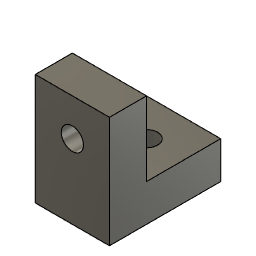
L_1.0 (Autodesk Fusion 360 design; units mm, degrees)
Autodesk Fusion 360 part; units mm, degrees
sketch "Sketch1" plane through (0, 0, 0) normal (0, 1, 0) x (1, 0, 0)
  line L0 (0, 0) -> (10, 0)
  line L1 (5, 0) -> (5, 10)
  line L2 (0, 0) -> (0, 15)
  line L3 (0, 15) -> (10, 15)
  line L4 (10, 15) -> (10, 0)
  circle A0 centre (5, 10) radius 1.5
  dimension "d1" = 3
  constraint coincident L0.start L2.start
  constraint horizontal L0
  constraint midpoint L0 L1.start
  constraint perpendicular L0 L1
  constraint perpendicular L0 L2
  constraint perpendicular L2 L3
  constraint perpendicular L0 L4
  constraint coincident L1.end A0.centre
  measures "d1" diameter of A0
extrude "Extrude1" add sketch "Sketch1" along normal blind 5
sketch "Sketch2" plane through (0, 0, 0) normal (0, 0, 1) x (1, 0, 0)
  line L0 (0, 0) -> (10, 0)
  line L1 (10, 0) -> (10, 5)
  line L2 (10, 5) -> (0, 5)
  line L3 (0, 5) -> (0, 0)
  line L4 (5, 0) -> (5, 10)
  line L5 (0, 5) -> (0, 15)
  line L6 (0, 15) -> (10, 15)
  line L7 (10, 15) -> (10, 5)
  circle A0 centre (5, 10) radius 1.5
  dimension "d4" = 10
  dimension "d5" = 3
  constraint midpoint L0 L4.start
  constraint perpendicular L2 L4
  constraint coincident L2.end L3.start
  constraint perpendicular L2 L5
  constraint perpendicular L5 L6
  constraint coincident L1.end L2.start
  constraint perpendicular L2 L7
  constraint coincident L4.end A0.centre
  measures "d4" distance of L4.start L4.end
  measures "d5" diameter of A0
extrude "Extrude2" add sketch "Sketch2" against normal blind 5 contours L2 L5 L6 L7
